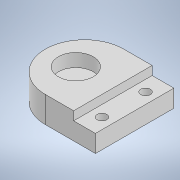
# Autodesk Inventor part: Деталь основы рулевого управления
Saved by Autodesk Inventor 2020 (Build 240168000, 168)
## iProperties
Created: 2021-06-17
Part Number: Деталь основы рулевого управления
Material: Типовые
Document SubType Name: Modeling
Designer: Антон
Density: 1 g/cm^3
Appearance: По умолчанию
Author: Антон
Autodesk Inventor part; units mm, degrees
ref_plane "YZ Plane" through (0, 0, 0) normal (1, 0, 0) x (0, 1, 0)
ref_plane "XZ Plane" through (0, 0, 0) normal (0, 1, 0) x (-1, 0, 0)
ref_plane "XY Plane" through (0, 0, 0) normal (0, 0, 1) x (1, 0, 0)
sketch "Эскиз1" plane through (0, 0, 0) normal (0, 1, 0) x (-1, 0, 0)
  line L0 (0, 0) -> (20.5, 0)
  line L1 (20.5, 0) -> (20.5, -18)
  line L2 (20.5, -18) -> (0, -18)
  line L3 (0, -18) -> (0, 0)
  dimension "d0" = 20.5
  dimension "d1" = 18
  constraints: 8 end point, 2 parallel, 1 horizontal, 1 perpendicular
  measures "d0" distance of L1.end L2.end
  measures "d1" distance of L0.end L1.end
extrude "Выдавливание1" add sketch "Эскиз1" along normal blind 6
sketch "Эскиз2" plane through (0, 6, 0) normal (0, 1, 0) x (1, 0, 0)
  line L0 (-20.5, 18) -> (-20.5, 0) projected
  line L1 (-20.5, 9) -> (-13.5, 9)
  circle A0 centre (-13.5, 9) radius 4
  point P0 (0, 0)
  dimension "d4" = 7
  dimension "d5" = 8
  constraints: 2 end point, 1 centre point, 1 coincident, 1 horizontal, 1 midpoint
  measures "d4" distance of L1.start L1.end
  measures "d5" diameter of A0
extrude "Выдавливание2" cut sketch "Эскиз2" against normal blind 3
fillet "Сопряжение1" radius 9 2 edges at (-20.5, 3, 0) (-20.5, 3, -18)
sketch "Эскиз3" plane through (0, 0, 0) normal (0, -1, 0) x (1, 0, 0)
  line L0 (0, 0) -> (0, -18) projected
  line L1 (0, -9) -> (-2.5, -9)
  line L2 (-2.5, -4) -> (-2.5, -14)
  dimension "d9" = 2.5
  dimension "d10" = 10
  constraints: 4 end point, 2 midpoint, 1 horizontal, 1 perpendicular
  measures "d9" distance of L1.end L1.start
  measures "d10" distance of L2.start L2.end
hole "Отверстие1" at (-2.5, 0, -4) at (-2.5, 0, -14) direction (0, 1, 0) diameter 2.2 end through all countersink diameter 3.9 countersink angle 90
sketch "Эскиз4" plane through (0, 6, 0) normal (0, 1, 0) x (1, 0, 0)
  line L0 (0, 0) -> (-5, 0)
  line L1 (-5, 0) -> (-5, 18)
  line L2 (-5, 18) -> (0, 18)
  line L3 (0, 18) -> (0, 0)
  line L4 (0, 18) -> (-11.5, 18) projected
  dimension "d18" = 5
  constraints: 8 end point, 2 parallel, 1 collinear, 1 horizontal, 1 perpendicular
  measures "d18" distance between parallel lines of L3 L1
extrude "Выдавливание3" cut sketch "Эскиз4" against normal blind 2
